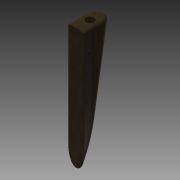
# Autodesk Inventor part: Version 1
Saved by Autodesk Inventor 2015 SP2 (Build 190223200, 223)
## iProperties
Created: 2016-03-30
Part Number: Version 1
Material: Wood (Maple)
Document SubType Name: Modeling
Designer: cvhssub1
Density: 0.67 g/cm^3
Appearance: Natural Maple - Glossy Dark Tint
Author: cvhssub1
Autodesk Inventor part; units mm, degrees
ref_plane "YZ Plane" through (0, 0, 0) normal (1, 0, 0) x (0, 1, 0)
ref_plane "XZ Plane" through (0, 0, 0) normal (0, 1, 0) x (-1, 0, 0)
ref_plane "XY Plane" through (0, 0, 0) normal (0, 0, 1) x (1, 0, 0)
sketch "Sketch2" plane through (0, 0, 0) normal (1, 0, 0) x (0, 1, 0)
  line L0 (0, 0) -> (70, 0)
  line L1 (0, 0) -> (0, -305)
  line L2 (0, -305) -> (20, -305)
  line L3 (20, -305) -> (70, 0)
  dimension "d2" = 70
  dimension "d3" = 305
  dimension "d4" = 20
  constraints: 8 end point, 1 horizontal, 1 perpendicular, 1 vertical
  measures "d2" distance of L0.start L0.end
  measures "d3" distance of L0.start L1.end
  measures "d4" distance of L1.end L2.end
extrude "Extrusion1" add sketch "Sketch2" along normal blind 40
sketch "Sketch3" plane through (0, 0, 0) normal (0, 0, 1) x (1, 0, 0)
  line L0 (0, 35) -> (40, 35)
  line L1 (0, 0) -> (40, 0) projected
  line L2 (20, 0) -> (20, 70)
  line L3 (0, 70) -> (40, 70) projected
  circle A0 centre (20, 35) radius 10
  dimension "d7" = 35
  dimension "d8" = 20
  constraints: 4 end point, 3 midpoint, 1 centre point
  measures "d7" distance of L1.start L0.start
  measures "d8" diameter of A0
extrude "Extrusion2" cut sketch "Sketch3" against normal blind 52
fillet "Fillet1" radius 300 1 edges at (20, 20, -305)
full round fillet "Fillet6" first side at (40, 35.5964, -67.5289) centre faces at (26.6667, 58.9297, -67.5289) second side at (0, 35.5964, -67.5289)
fillet "Fillet7" radius 5 5 edges at (40, 24.8666, 0) (0, 24.8666, 0) (5.8578, 64.064, 0) (20, 70, 0) (34.1422, 64.064, 0)
fillet "Fillet8" radius 1 8 edges at (38.5355, 0, -1.4645) (40, 0, -132.406) (20, 0, -305) (36.6848, 0, -286.2736) (3.3152, 0, -286.2736) (0, 0, -132.406) (1.4645, 0, -1.4645) (20, 0, 0)
body "Solid1"
